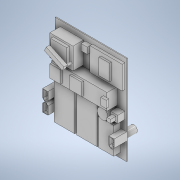
# Autodesk Inventor part: БАСУ
Saved by Autodesk Inventor 2022 (Build 260153000, 153)
## iProperties
Created: 2022-05-03
Part Number: БАСУ
Material: Пластик АБС
Document SubType Name: Modeling
Designer: Кочетов.А.И.
Density: 1.06 g/cm^3
Appearance: Алюминий — темный
Author: Кочетов.А.И.
Autodesk Inventor part; units mm, degrees
ref_plane "YZ Plane" through (0, 0, 0) normal (1, 0, 0) x (0, 1, 0)
ref_plane "XZ Plane" through (0, 0, 0) normal (0, 1, 0) x (-1, 0, 0)
ref_plane "XY Plane" through (0, 0, 0) normal (0, 0, 1) x (1, 0, 0)
sketch "Эскиз1" plane through (0, 0, 0) normal (0, 0, 1) x (1, 0, 0)
  line L0 (-40, -50) -> (40, -50)
  line L1 (40, -50) -> (40, 50)
  line L2 (40, 50) -> (-40, 50)
  line L3 (-40, 50) -> (-40, -50)
  line L4 (-40, -50) -> (40, 50) construction
  line L5 (40, -50) -> (-40, 50) construction
  point P0 (0, 0)
  dimension "d0" = 100
  dimension "d1" = 80
  constraints: 12 end point, 2 midpoint, 2 parallel, 1 horizontal, 1 perpendicular
  measures "d0" distance of L0.end L1.end
  measures "d1" distance of L1.end L2.end
extrude "Выдавливание1" add sketch "Эскиз1" along normal blind 0.5 and the other way blind 0.5
sketch "Эскиз2" plane through (0, 0, 0.5) normal (0, 0, 1) x (1, 0, 0)
  line L0 (40, -21) -> (34, -21)
  line L1 (34, -21) -> (34, -32)
  line L2 (34, -32) -> (40, -32)
  line L3 (40, -32) -> (40, -21)
  line L4 (-40, 50) -> (-40, -50) projected
  line L5 (-40, -12) -> (-34, -12)
  line L6 (-34, -12) -> (-34, -23)
  line L7 (-34, -23) -> (-40, -23)
  line L8 (-40, -23) -> (-40, -12)
  line L9 (-40, -24) -> (-34, -24)
  line L10 (-34, -24) -> (-34, -35)
  line L11 (-34, -35) -> (-40, -35)
  line L12 (-40, -35) -> (-40, -24)
  line L13 (40, -50) -> (40, 50) projected
  line L14 (-40, -50) -> (40, -50) projected
  line L15 (-40, -26) -> (-38, -24)
  line L16 (-36, -24) -> (-34, -26)
  line L17 (-36, -23) -> (-34, -21)
  line L18 (-38, -23) -> (-40, -21)
  line L19 (38, -32) -> (40, -30)
  line L20 (36, -32) -> (34, -30)
  point P0 (0, 0)
  dimension "d7" = 11
  dimension "d8" = 6
  dimension "d9" = 15
  dimension "d10" = 1
  dimension "d11" = 18
  dimension "d12" = 45
  dimension "d13" = 2
  dimension "d14" = 2
  dimension "d15" = 45
  constraints: 36 end point, 15 point on line, 8 equal length, 7 perpendicular, 6 parallel, 3 horizontal
  measures "d7" distance of L0.end L1.end
  measures "d8" distance of L10.end L11.end
  measures "d9" distance between parallel lines of L14 L11
  measures "d10" distance between parallel lines of L7 L9
  measures "d11" distance between parallel lines of L14 L2
  measures "d12" angle of L2 L19
  measures "d13" horizontal distance of L19.end L19.start
  measures "d14" horizontal distance of L16.start L16.end
  measures "d15" angle of L9 L16
extrude "Выдавливание2" add sketch "Эскиз2" along normal blind 14 contours L3 L19 L2 L20 L1 L0 | L5 L6 L17 L7 L18 L4 | L15 L9 L16 L10 L11 L4
sketch "Эскиз3" plane through (0, 0, 14.5) normal (0, 0, 1) x (1, 0, 0)
  line L0 (-38, -23) -> (-36, -23) projected
  line L1 (-36, -23) -> (-34, -21) projected
  line L2 (-34, -21) -> (-34, -12) projected
  line L3 (-34, -12) -> (-40, -12) projected
  line L4 (-40, -12) -> (-40, -21) projected
  line L5 (-40, -21) -> (-38, -23) projected
  line L6 (-36, -24) -> (-38, -24) projected
  line L7 (-38, -24) -> (-40, -26) projected
  line L8 (-40, -26) -> (-40, -35) projected
  line L9 (-40, -35) -> (-34, -35) projected
  line L10 (-34, -35) -> (-34, -26) projected
  line L11 (-34, -26) -> (-36, -24) projected
  line L12 (36, -32) -> (38, -32) projected
  line L13 (38, -32) -> (40, -30) projected
  line L14 (40, -30) -> (40, -21) projected
  line L15 (40, -21) -> (34, -21) projected
  line L16 (34, -21) -> (34, -30) projected
  line L17 (34, -30) -> (36, -32) projected
  line L18 (-39.5, -12.5) -> (-34.5, -12.5)
  line L19 (-34.5, -12.5) -> (-34.5, -20.7929)
  line L20 (-34.5, -20.7929) -> (-36.2071, -22.5)
  line L21 (-36.2071, -22.5) -> (-37.7929, -22.5)
  line L22 (-37.7929, -22.5) -> (-39.5, -20.7929)
  line L23 (-39.5, -20.7929) -> (-39.5, -12.5)
  line L24 (-40, -50) -> (-40, 50) projected
  line L25 (-39.5, -34.5) -> (-34.5, -34.5)
  line L26 (-34.5, -34.5) -> (-34.5, -26.2071)
  line L27 (-34.5, -26.2071) -> (-36.2071, -24.5)
  line L28 (-36.2071, -24.5) -> (-37.7929, -24.5)
  line L29 (-37.7929, -24.5) -> (-39.5, -26.2071)
  line L30 (-39.5, -26.2071) -> (-39.5, -34.5)
  line L31 (34.5, -21.5) -> (39.5, -21.5)
  line L32 (39.5, -21.5) -> (39.5, -29.7929)
  line L33 (39.5, -29.7929) -> (37.7929, -31.5)
  line L34 (37.7929, -31.5) -> (36.2071, -31.5)
  line L35 (36.2071, -31.5) -> (34.5, -29.7929)
  line L36 (34.5, -29.7929) -> (34.5, -21.5)
  line L37 (34, -30) -> (36, -32) projected
  line L38 (38, -32) -> (40, -30) projected
  point P0 (0, 0)
  dimension "d18" = 0.5
  dimension "d19" = 0.5
  dimension "d20" = 0.5
  dimension "d23" = 0.5
  dimension "d24" = 0.5
  dimension "d26" = 0.5
  dimension "d27" = 0.5
  dimension "d28" = 0.5
  dimension "d29" = 0.5
  dimension "d30" = 0.5
  dimension "d32" = 0.5
  dimension "d33" = 0.5
  dimension "d34" = 0.5
  dimension "d35" = 0.5
  dimension "d36" = 0.5
  dimension "d37" = 0.5
  dimension "d38" = 0.5
  dimension "d39" = 0.5
  constraints: 36 end point, 7 parallel, 6 perpendicular, 3 horizontal
  measures "d18" distance between parallel lines of L3 L18
  measures "d19" distance between parallel lines of L2 L19
  measures "d20" distance between parallel lines of L4 L23
  measures "d23" distance between parallel lines of L1 L20
  measures "d24" distance between parallel lines of L5 L22
  measures "d26" distance between parallel lines of L10 L26
  measures "d27" distance between parallel lines of L8 L30
  measures "d28" distance between parallel lines of L9 L25
  measures "d29" distance between parallel lines of L7 L29
  measures "d30" distance between parallel lines of L11 L27
  measures "d32" distance between parallel lines of L0 L21
  measures "d33" distance between parallel lines of L6 L28
  measures "d34" distance between parallel lines of L17 L35
  measures "d35" distance between parallel lines of L13 L33
  measures "d36" distance between parallel lines of L12 L34
  measures "d37" distance between parallel lines of L16 L36
  measures "d38" distance between parallel lines of L14 L32
  measures "d39" distance between parallel lines of L15 L31
extrude "Выдавливание3" cut sketch "Эскиз3" against normal blind 8 contours L18 L19 L20 L21 L22 L23 | L30 L29 L28 L27 L26 L25 | L31 L32 L33 L34 L35 L36
sketch "Эскиз4" plane through (0, 0, 6.5) normal (0, 0, 1) x (1, 0, 0)
  line L0 (-37.7929, -22.5) -> (-39.5, -20.7929) projected
  line L1 (-36.2071, -22.5) -> (-37.7929, -22.5) projected
  line L2 (-34.5, -20.7929) -> (-36.2071, -22.5) projected
  line L3 (-34.5, -12.5) -> (-34.5, -20.7929) projected
  line L4 (-39.5, -12.5) -> (-34.5, -12.5) projected
  line L5 (-39.5, -20.7929) -> (-39.5, -12.5) projected
  line L6 (-34.5, -26.2071) -> (-34.5, -34.5) projected
  line L7 (-36.2071, -24.5) -> (-34.5, -26.2071) projected
  line L8 (-37.7929, -24.5) -> (-36.2071, -24.5) projected
  line L9 (-39.5, -26.2071) -> (-37.7929, -24.5) projected
  line L10 (-39.5, -34.5) -> (-39.5, -26.2071) projected
  line L11 (-34.5, -34.5) -> (-39.5, -34.5) projected
  line L12 (36.2071, -31.5) -> (34.5, -29.7929) projected
  line L13 (37.7929, -31.5) -> (36.2071, -31.5) projected
  line L14 (39.5, -29.7929) -> (37.7929, -31.5) projected
  line L15 (39.5, -21.5) -> (39.5, -29.7929) projected
  line L16 (34.5, -21.5) -> (39.5, -21.5) projected
  line L17 (34.5, -29.7929) -> (34.5, -21.5) projected
  circle A0 centre (-37, -20.5) radius 1
  circle A1 centre (-37, -14.5) radius 1
  line L18 (-39.5, -12.5) -> (-34.5, -12.5) construction
  line L19 (-37, -12.5) -> (-37, -34.5) construction
  line L20 (-34.5, -34.5) -> (-39.5, -34.5) construction
  circle A2 centre (-37, -26.5) radius 1
  circle A3 centre (-37, -32.5) radius 1
  line L21 (34.5, -21.5) -> (39.5, -21.5) construction
  line L22 (37, -21.5) -> (37, -31.5) construction
  circle A4 centre (37, -23.5) radius 1
  circle A5 centre (37, -29.5) radius 1
  point P0 (0, 0)
  dimension "d42" = 6
  dimension "d43" = 2
  dimension "d44" = 2
  dimension "d45" = 6
  dimension "d46" = 2
  dimension "d47" = 2
  dimension "d48" = 2
  dimension "d49" = 2
  dimension "d50" = 6
  dimension "d51" = 2
  constraints: 6 centre point, 6 point on line, 4 end point, 4 midpoint, 2 equal radius
  measures "d42" distance of A0.centre A1.centre
  measures "d43" diameter of A2
  measures "d44" diameter of A3
  measures "d45" distance of A3.centre A2.centre
  measures "d46" distance from line of L4 A1.centre
  measures "d47" distance from line of L11 A3.centre
  measures "d48" diameter of A4
  measures "d49" diameter of A5
  measures "d50" distance of A4.centre A5.centre
  measures "d51" distance from line of L16 A4.centre
extrude "Выдавливание4" add sketch "Эскиз4" along normal blind 6 contours A0 | A1 | A2 | A3 | A4 | A5
sketch "Эскиз5" plane through (0, 0, 0.5) normal (0, 0, 1) x (1, 0, 0)
  line L0 (-33, -2) -> (-10, -2)
  line L1 (-10, -2) -> (-10, -44)
  line L2 (-10, -44) -> (-33, -44)
  line L3 (-33, -44) -> (-33, -2)
  line L4 (-8, -2) -> (15, -2)
  line L5 (15, -2) -> (15, -44)
  line L6 (15, -44) -> (-8, -44)
  line L7 (-8, -44) -> (-8, -2)
  line L8 (-40, -50) -> (40, -50) projected
  line L9 (-40, -35) -> (-40, -50) projected
  line L10 (16.5, -44) -> (33.5, -44)
  line L11 (33.5, -44) -> (33.5, -14)
  line L12 (33.5, -14) -> (16.5, -14)
  line L13 (16.5, -14) -> (16.5, -44)
  point P0 (0, 0)
  dimension "d54" = 42
  dimension "d55" = 23
  dimension "d56" = 48
  dimension "d59" = 55
  dimension "d60" = 48
  dimension "d63" = 1.5
  dimension "d64" = 17
  dimension "d65" = 36
  constraints: 24 end point, 6 parallel, 3 horizontal, 3 perpendicular, 2 equal length, 2 point on line
  measures "d54" distance between parallel lines of L6 L4
  measures "d55" distance of L1.end L2.end
  measures "d56" distance between parallel lines of L8 L0
  measures "d59" distance between parallel lines of L9 L5
  measures "d60" distance between parallel lines of L3 L5
  measures "d63" distance between parallel lines of L5 L13
  measures "d64" distance of L10.start L10.end
  measures "d65" distance between parallel lines of L8 L12
extrude "Выдавливание5" add sketch "Эскиз5" along normal blind 8
sketch "Эскиз6" plane through (0, 0, -0.5) normal (0, 0, -1) x (-1, 0, 0)
  line L0 (-32, -23) -> (12, -23)
  line L1 (12, -23) -> (12, -45)
  line L2 (12, -45) -> (-32, -45)
  line L3 (-32, -45) -> (-32, -23)
  line L4 (-40, -50) -> (40, -50) projected
  line L5 (-40, 50) -> (-40, -50) projected
  point P0 (0, 0)
  dimension "d66" = 44
  dimension "d67" = 22
  dimension "d68" = 5
  dimension "d69" = 8
  constraints: 8 end point, 2 parallel, 1 horizontal, 1 perpendicular
  measures "d66" distance of L0.start L0.end
  measures "d67" distance of L0.end L1.end
  measures "d68" distance between parallel lines of L4 L2
  measures "d69" distance between parallel lines of L5 L3
extrude "Выдавливание6" add sketch "Эскиз6" along normal blind 8
sketch "Эскиз7" plane through (0, 0, -0.5) normal (0, 0, -1) x (-1, 0, 0)
  line L0 (23, -25) -> (33, -25)
  line L1 (33, -25) -> (33, -32)
  line L2 (33, -32) -> (23, -32)
  line L3 (23, -32) -> (23, -25)
  line L4 (23, -11) -> (33, -11)
  line L5 (33, -11) -> (33, -18)
  line L6 (33, -18) -> (23, -18)
  line L7 (23, -18) -> (23, -11)
  line L8 (-40, -50) -> (40, -50) projected
  line L9 (40, -50) -> (40, 50) projected
  point P0 (0, 0)
  point P1 (33, -14.5)
  dimension "d72" = 7
  dimension "d73" = 10
  dimension "d74" = 7
  dimension "d75" = 18
  dimension "d76" = 7
  constraints: 16 end point, 4 parallel, 2 equal length, 2 horizontal, 2 perpendicular, 1 midpoint, 1 vertical alignment
  measures "d72" distance of L0.end L1.end
  measures "d73" distance of L1.end L2.end
  measures "d74" distance between parallel lines of L0 L6
  measures "d75" distance between parallel lines of L8 L2
  measures "d76" distance between parallel lines of L9 L1
extrude "Выдавливание7" add sketch "Эскиз7" along normal blind 3
sketch "Эскиз8" plane through (0, 0, -8.5) normal (0, 0, -1) x (-1, 0, 0)
  circle A0 centre (-28, -34) radius 4
  circle A1 centre (8, -34) radius 4
  line L0 (-32, -45) -> (-32, -23) construction
  line L1 (-32, -34) -> (12, -34) construction
  line L2 (12, -23) -> (12, -45) construction
  line L3 (12, -45) -> (12, -23) construction
  line L4 (-32, -23) -> (-32, -45) construction
  point P0 (0, 0)
  dimension "d79" = 8
  constraints: 2 centre point, 2 end point, 2 midpoint, 2 tangent, 1 equal radius, 1 horizontal alignment, 1 point on line
  measures "d79" diameter of A0
extrude "Выдавливание8" add sketch "Эскиз8" along normal blind 11
sketch "Эскиз9" plane through (0, 0, -8.5) normal (0, 0, -1) x (-1, 0, 0)
  line L0 (2, -44) -> (-11, -44)
  line L1 (-11, -44) -> (-11, -31)
  line L2 (-11, -31) -> (2, -31)
  line L3 (2, -31) -> (2, -44)
  line L4 (12, -34) -> (12, -23) projected
  line L5 (-32, -45) -> (12, -45) projected
  point P0 (0, 0)
  dimension "d82" = 13
  dimension "d83" = 10
  dimension "d84" = 1
  constraints: 8 end point, 2 parallel, 2 perpendicular, 1 horizontal
  measures "d82" distance of L0.start L0.end
  measures "d83" distance between parallel lines of L4 L3
  measures "d84" distance between parallel lines of L5 L0
extrude "Выдавливание9" add sketch "Эскиз9" along normal blind 8
sketch "Эскиз10" plane through (0, 0, -8.5) normal (0, 0, -1) x (-1, 0, 0)
  line L0 (-8, -25) -> (2, -25)
  line L1 (2, -25) -> (2, -29)
  line L2 (2, -29) -> (-8, -29)
  line L3 (-8, -29) -> (-8, -25)
  line L4 (12, -23) -> (-32, -23) projected
  line L5 (12, -34) -> (12, -23) projected
  point P0 (0, 0)
  dimension "d87" = 10
  dimension "d88" = 4
  dimension "d89" = 2
  dimension "d90" = 10
  constraints: 8 end point, 2 parallel, 1 horizontal, 1 perpendicular
  measures "d87" distance of L0.start L0.end
  measures "d88" distance of L2.end L0.start
  measures "d89" distance between parallel lines of L4 L0
  measures "d90" distance between parallel lines of L5 L1
extrude "Выдавливание10" add sketch "Эскиз10" along normal blind 10
sketch "Эскиз11" plane through (0, 0, -18.5) normal (0, 0, -1) x (-1, 0, 0)
  circle A0 centre (-7, -26) radius 1
  line L0 (-8, -29) -> (2, -29) projected
  line L1 (2, -29) -> (2, -25) projected
  line L2 (2, -25) -> (-8, -25) projected
  line L3 (-8, -25) -> (-8, -29) projected
  line L4 (2, -25) -> (-8, -25) projected
  line L5 (-8, -25) -> (-8, -29) projected
  point P0 (0, 0)
  dimension "d93" = 2
  constraints: 2 tangent, 1 centre point
  measures "d93" diameter of A0
extrude "Выдавливание11" add sketch "Эскиз11" along normal blind 1 contours A0
sketch "Эскиз12" plane through (0, 0, -8.5) normal (0, 0, -1) x (-1, 0, 0)
  line L0 (-22, -25) -> (-12, -25)
  line L1 (-12, -25) -> (-12, -41)
  line L2 (-12, -41) -> (-22, -41)
  line L3 (-22, -41) -> (-22, -25)
  line L4 (12, -23) -> (-32, -23) projected
  line L5 (-32, -23) -> (-32, -34) projected
  point P0 (0, 0)
  dimension "d96" = 10
  dimension "d97" = 16
  dimension "d98" = 2
  dimension "d99" = 10
  constraints: 8 end point, 2 parallel, 1 horizontal, 1 perpendicular
  measures "d96" distance of L0.start L0.end
  measures "d97" distance of L2.end L0.start
  measures "d98" distance between parallel lines of L4 L0
  measures "d99" distance between parallel lines of L5 L3
extrude "Выдавливание12" add sketch "Эскиз12" along normal blind 5
sketch "Эскиз13" plane through (0, 0, 0.5) normal (0, 0, 1) x (1, 0, 0)
  point P0 (0, 0)
sketch "Эскиз14" plane through (0, 0, 0.5) normal (0, 0, 1) x (1, 0, 0)
  circle A0 centre (23, -7) radius 6
  line L0 (40, -21) -> (40, 50) projected
  line L1 (-40, -50) -> (40, -50) projected
  point P0 (0, 0)
  dimension "d102" = 12
  dimension "d103" = 17
  dimension "d104" = 43
  constraints: 1 centre point
  measures "d102" diameter of A0
  measures "d103" distance from line of L0 A0.centre
  measures "d104" distance from line of L1 A0.centre
extrude "Выдавливание13" add sketch "Эскиз14" along normal blind 10
sketch "Эскиз15" plane through (0, 0, 0.5) normal (0, 0, 1) x (1, 0, 0)
  line L0 (30, -2) -> (38, -2)
  line L1 (38, -2) -> (38, -10)
  line L2 (38, -10) -> (30, -10)
  line L3 (30, -10) -> (30, -2)
  line L4 (-40, -50) -> (40, -50) projected
  line L5 (40, -21) -> (40, 50) projected
  point P0 (0, 0)
  dimension "d107" = 8
  dimension "d108" = 48
  dimension "d109" = 2
  constraints: 8 end point, 2 parallel, 2 perpendicular, 1 horizontal
  measures "d107" distance of L0.start L0.end
  measures "d108" distance between parallel lines of L4 L0
  measures "d109" distance between parallel lines of L5 L1
extrude "Выдавливание14" add sketch "Эскиз15" along normal blind 8
sketch "Эскиз16" plane through (0, 0, 8.5) normal (0, 0, 1) x (1, 0, 0)
  line L0 (32, -4) -> (36, -4)
  line L1 (36, -4) -> (36, -8)
  line L2 (36, -8) -> (32, -8)
  line L3 (32, -8) -> (32, -4)
  line L4 (30, -10) -> (38, -10) projected
  line L5 (38, -10) -> (38, -2) projected
  line L6 (38, -2) -> (30, -2) projected
  line L7 (30, -2) -> (30, -10) projected
  point P0 (0, 0)
  dimension "d115" = 4
  dimension "d116" = 2
  dimension "d117" = 2
  constraints: 8 end point, 2 parallel, 2 perpendicular, 1 horizontal
  measures "d115" distance of L0.end L1.end
  measures "d116" distance between parallel lines of L5 L1
  measures "d117" distance between parallel lines of L6 L0
extrude "Выдавливание15" add sketch "Эскиз16" along normal blind 6 contours L0 L1 L2 L3
sketch "Эскиз17" plane through (0, 0, 0.5) normal (0, 0, 1) x (1, 0, 0)
  line L0 (-32, 18) -> (30, 18)
  line L1 (30, 18) -> (30, 0)
  line L2 (30, 0) -> (-32, 0)
  line L3 (-32, 0) -> (-32, 18)
  line L4 (40, -21) -> (40, 50) projected
  line L5 (40, 50) -> (-40, 50) projected
  point P0 (0, 0)
  dimension "d120" = 18
  dimension "d121" = 62
  dimension "d122" = 10
  dimension "d123" = 32
  constraints: 8 end point, 2 parallel, 1 horizontal, 1 perpendicular
  measures "d120" distance of L0.end L1.end
  measures "d121" distance of L0.start L0.end
  measures "d122" distance between parallel lines of L4 L1
  measures "d123" distance between parallel lines of L5 L0
extrude "Выдавливание16" add sketch "Эскиз17" along normal blind 12
sketch "Эскиз18" plane through (0, 0, 12.5) normal (0, 0, 1) x (1, 0, 0)
  line L0 (-10, 16) -> (4, 16)
  line L1 (4, 16) -> (4, 2)
  line L2 (4, 2) -> (-10, 2)
  line L3 (-10, 2) -> (-10, 16)
  line L4 (-32, 18) -> (-32, 0) projected
  line L5 (-32, 16) -> (-20, 16)
  line L6 (-20, 16) -> (-20, 2)
  line L7 (-20, 2) -> (-32, 2)
  line L8 (-32, 2) -> (-32, 16)
  line L9 (30, 18) -> (-32, 18) projected
  point P0 (0, 0)
  dimension "d126" = 14
  dimension "d127" = 14
  dimension "d128" = 2
  dimension "d129" = 2
  dimension "d130" = 12
  dimension "d131" = 22
  constraints: 16 end point, 4 parallel, 3 perpendicular, 2 horizontal, 1 point on line
  measures "d126" distance of L5.end L6.end
  measures "d127" distance of L0.end L1.end
  measures "d128" distance between parallel lines of L9 L0
  measures "d129" distance between parallel lines of L9 L5
  measures "d130" distance between parallel lines of L4 L6
  measures "d131" distance between parallel lines of L4 L3
extrude "Выдавливание17" add sketch "Эскиз18" along normal blind 2
sketch "Эскиз19" plane through (0, 0, 12.5) normal (0, 0, 1) x (1, 0, 0)
  line L0 (26, 13) -> (32, 13)
  line L1 (32, 13) -> (32, 5)
  line L2 (32, 5) -> (26, 5)
  line L3 (26, 5) -> (26, 13)
  line L4 (30, 0) -> (30, 18) projected
  line L5 (-32, 0) -> (30, 0) projected
  point P0 (0, 0)
  dimension "d134" = 6
  dimension "d135" = 8
  dimension "d136" = 2
  dimension "d137" = 5
  constraints: 8 end point, 2 parallel, 1 horizontal, 1 perpendicular
  measures "d134" distance of L0.start L0.end
  measures "d135" distance of L0.end L1.end
  measures "d136" distance between parallel lines of L4 L1
  measures "d137" distance between parallel lines of L5 L2
extrude "Выдавливание18" add sketch "Эскиз19" along normal blind 3
sketch "Эскиз20" plane through (0, 0, 0.5) normal (0, 0, 1) x (1, 0, 0)
  line L0 (-34, 44) -> (-8, 44)
  line L1 (-8, 44) -> (-8, 20)
  line L2 (-8, 20) -> (-34, 20)
  line L3 (-34, 20) -> (-34, 44)
  line L4 (40, 50) -> (-40, 50) projected
  line L5 (-40, 50) -> (-40, -12) projected
  point P0 (0, 0)
  dimension "d140" = 26
  dimension "d141" = 24
  dimension "d142" = 6
  dimension "d143" = 6
  constraints: 8 end point, 2 parallel, 1 horizontal, 1 perpendicular
  measures "d140" distance of L0.start L0.end
  measures "d141" distance of L2.end L0.start
  measures "d142" distance between parallel lines of L4 L0
  measures "d143" distance between parallel lines of L5 L3
extrude "Выдавливание19" add sketch "Эскиз20" along normal blind 12
sketch "Эскиз21" plane through (0, 0, 12.5) normal (0, 0, 1) x (1, 0, 0)
  line L0 (-23, 25) -> (-15, 25)
  line L1 (-15, 25) -> (-15, 21)
  line L2 (-15, 21) -> (-23, 21)
  line L3 (-23, 21) -> (-23, 25)
  line L4 (-30, 42) -> (-12, 42)
  line L5 (-12, 42) -> (-12, 26)
  line L6 (-12, 26) -> (-30, 26)
  line L7 (-30, 26) -> (-30, 42)
  line L8 (-8, 20) -> (-8, 44) projected
  line L9 (-8, 44) -> (-34, 44) projected
  line L10 (-34, 20) -> (-8, 20) projected
  point P0 (0, 0)
  dimension "d146" = 18
  dimension "d147" = 4
  dimension "d148" = 2
  dimension "d149" = 16
  dimension "d150" = 8
  dimension "d151" = 4
  dimension "d152" = 7
  dimension "d153" = 1
  constraints: 16 end point, 4 parallel, 2 horizontal, 2 perpendicular
  measures "d146" distance of L4.start L4.end
  measures "d147" distance between parallel lines of L8 L5
  measures "d148" distance between parallel lines of L4 L9
  measures "d149" distance between parallel lines of L4 L6
  measures "d150" distance of L1.end L2.end
  measures "d151" distance of L0.end L1.end
  measures "d152" distance between parallel lines of L8 L1
  measures "d153" distance between parallel lines of L10 L2
extrude "Выдавливание20" add sketch "Эскиз21" along normal blind 3
sketch "Эскиз22" plane through (0, 0, 12.5) normal (0, 0, 1) x (1, 0, 0)
  circle A0 centre (-10, 27) radius 1
  line L0 (-8, 20) -> (-8, 44) projected
  line L1 (-34, 20) -> (-8, 20) projected
  point P0 (0, 0)
  dimension "d156" = 2
  dimension "d157" = 2
  dimension "d158" = 7
  constraints: 1 centre point
  measures "d156" diameter of A0
  measures "d157" distance from line of L0 A0.centre
  measures "d158" distance from line of L1 A0.centre
extrude "Выдавливание21" add sketch "Эскиз22" along normal blind 6
sketch "Эскиз23" plane through (-10, 27, 18.5) normal (0, 0, 1) x (1, 0, 0)
  line L0 (-17.9759, 11.1408) -> (1.9629, 1.8432)
  line L1 (1.9629, 1.8432) -> (-0.1502, -2.6884)
  line L2 (-0.1502, -2.6884) -> (-20.089, 6.6092)
  line L3 (-20.089, 6.6092) -> (-17.9759, 11.1408)
  circle A0 centre (0, 0) radius 1 construction
  line L4 (-24, -7) -> (2, -7) projected
  point P0 (10, -27)
  point P1 (0.9063, -0.4226)
  dimension "d161" = 5
  dimension "d162" = 22
  dimension "d163" = 2.5
  dimension "d164" = 25
  constraints: 8 end point, 2 parallel, 1 perpendicular, 1 tangent
  measures "d161" distance of L2.end L0.start
  measures "d162" distance of L0.start L0.end
  measures "d163" distance from line of L0 A0.centre
  measures "d164" angle of L4 L0
extrude "Выдавливание22" add sketch "Эскиз23" along normal blind 4
sketch "Эскиз24" plane through (0, 0, 0.5) normal (0, 0, 1) x (1, 0, 0)
  line L0 (-6, 44) -> (1, 44)
  line L1 (1, 44) -> (1, 37)
  line L2 (1, 37) -> (-6, 37)
  line L3 (-6, 37) -> (-6, 44)
  line L4 (40, 50) -> (-40, 50) projected
  line L5 (-40, 50) -> (-40, -12) projected
  point P0 (0, 0)
  dimension "d167" = 7
  dimension "d168" = 6
  dimension "d169" = 34
  constraints: 8 end point, 2 parallel, 2 perpendicular, 1 horizontal
  measures "d167" distance of L0.start L0.end
  measures "d168" distance between parallel lines of L4 L0
  measures "d169" distance between parallel lines of L5 L3
extrude "Выдавливание23" add sketch "Эскиз24" along normal blind 5
sketch "Эскиз25" plane through (0, 0, 0.5) normal (0, 0, 1) x (1, 0, 0)
  line L0 (2, 45) -> (38, 45)
  line L1 (38, 45) -> (38, 19)
  line L2 (38, 19) -> (2, 19)
  line L3 (2, 19) -> (2, 45)
  line L4 (40, 50) -> (-40, 50) projected
  line L5 (40, -21) -> (40, 50) projected
  point P0 (0, 0)
  dimension "d172" = 36
  dimension "d173" = 26
  dimension "d174" = 5
  dimension "d175" = 2
  constraints: 8 end point, 2 parallel, 1 horizontal, 1 perpendicular
  measures "d172" distance of L0.start L0.end
  measures "d173" distance between parallel lines of L2 L0
  measures "d174" distance between parallel lines of L0 L4
  measures "d175" distance between parallel lines of L5 L1
extrude "Выдавливание24" add sketch "Эскиз25" along normal blind 3
sketch "Эскиз26" plane through (0, 0, 3.5) normal (0, 0, 1) x (1, 0, 0)
  line L0 (14, 41) -> (26, 41)
  line L1 (26, 41) -> (26, 23)
  line L2 (26, 23) -> (14, 23)
  line L3 (14, 23) -> (14, 41)
  line L4 (38, 45) -> (2, 45) projected
  line L5 (2, 45) -> (2, 19) projected
  point P0 (0, 0)
  dimension "d178" = 12
  dimension "d179" = 18
  dimension "d180" = 4
  dimension "d181" = 12
  constraints: 8 end point, 2 parallel, 1 horizontal, 1 perpendicular
  measures "d178" distance of L0.start L0.end
  measures "d179" distance of L0.end L1.end
  measures "d180" distance between parallel lines of L0 L4
  measures "d181" distance between parallel lines of L5 L3
extrude "Выдавливание25" add sketch "Эскиз26" along normal blind 2
